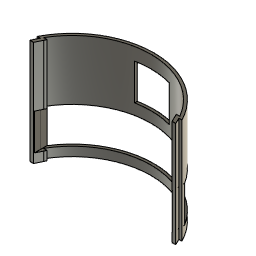
top cap pcb (Autodesk Fusion 360 design; units mm, degrees)
Autodesk Fusion 360 part; units mm, degrees
sketch "Sketch1" plane through (0, 0, 0) normal (0, 0, 1) x (1, 0, 0)
  arc A0 (40, 20.6155) -> (-40, 20.6155) centre (0, 0) ccw
  arc A1 (39.9116, 17.2383) -> (-40.1731, 16.7877) centre (-0.0351, 0.0189) ccw
  line L0 (-40, 20.6155) -> (-38.35, 20.6155)
  line L1 (40, 20.6155) -> (38.2797, 20.6155)
  line L2 (-40.1731, 16.7877) -> (-38.1731, 16.7877)
  line L3 (39.9116, 17.2383) -> (37.9116, 17.2383)
  line L4 (-36.35, 20.6155) -> (-38.1731, 16.7877)
  line L5 (36.2797, 20.6155) -> (37.9116, 17.2383)
  arc A2 (37.5794, 17.9258) -> (37.9116, 17.2383) centre (37.9116, 17.6623) ccw
  line L6 (35.69, 21.8359) -> (39.3471, 21.8359)
  line L7 (35.69, 21.8359) -> (36.2797, 20.6155)
  line L8 (-0.0351, 0.0189) -> (-0.0351, 49.45) construction
  line L9 (-35.7603, 21.8359) -> (-36.35, 20.6155)
  line L10 (-35.7603, 21.8359) -> (-39.4174, 21.8359)
  dimension "d2" = 80
  dimension "d4" = 2
  dimension "d5" = 2
  dimension "d6" = 2
  dimension "d7" = 2
  constraint coincident A1 L0.end
  constraint coincident A1 L1.end
  constraint horizontal L2
  constraint horizontal L3
  constraint coincident L5 A2.start
  constraint tangent L3 A2
  constraint coincident A0 L6.end
  constraint parallel L3 L6
  constraint parallel L5 L7
  constraint coincident A1.centre L8.start
  constraint vertical L8
  constraint symmetric L5.start L8 L4.start
  constraint symmetric L6.start L8 L9.start
  constraint symmetric L6.end L8 L10.end
  measures "d2" distance of A0.end A0.start
  measures "d4" distance of A1.end L2.end
  measures "d5" distance of A1.start L3.end
  measures "d6" distance of L0.end L4.start
  measures "d7" distance of L1.end L5.start
extrude "Extrude1" add sketch "Sketch1" along normal blind 58 contours A0 A1 L1 L6 | A0 A1 L6 L10 | A1 L3 L5 L6 L7 | A0 A1 L0 L10 | A1 L2 L4 L9 L10
sketch "Sketch2" plane through (0, 0, 0) normal (0, 1, 0) x (1, 0, 0)
  line L0 (0, 0) -> (0, -5)
  line L1 (0, -5) -> (38, -5)
  line L2 (38, -5) -> (-38, -5)
  line L3 (-38, -5) -> (-38, -25)
  line L4 (-38, -25) -> (38, -25)
  line L5 (38, -25) -> (38, -5)
  line L6 (-8.3, -51) -> (11.7, -51)
  line L7 (11.7, -51) -> (11.7, -31)
  line L8 (11.7, -31) -> (-8.3, -31)
  line L9 (-8.3, -31) -> (-8.3, -51)
  line L10 (-8.3, -51) -> (11.7, -31) construction
  line L11 (11.7, -51) -> (-8.3, -31) construction
  line L12 (0, -57.95) -> (0, -50.95)
  point P0 (1.7, -41)
  dimension "d10" = 5
  dimension "d11" = 38
  dimension "d12" = 76
  dimension "d13" = 20
  dimension "d14" = 20
  dimension "d15" = 20
  dimension "d16" = 7
  constraint coincident L0.start origin
  constraint vertical L0
  constraint perpendicular L0 L1
  constraint horizontal L2
  constraint vertical L3
  constraint horizontal L4
  constraint vertical L5
  constraint horizontal L6
  constraint perpendicular L6 L7
  constraint parallel L6 L8
  constraint parallel L7 L9
  constraint coincident L10 P0
  constraint coincident L11 P0
  constraint perpendicular L4 L12
  measures "d10" distance of L0.start L0.end
  measures "d11" distance of L0.end L1.end
  measures "d12" distance of L1.end L2.end
  measures "d13" distance of L1.end L4.end
  measures "d14" distance of L7.end L8.end
  measures "d15" distance of L6.end L7.end
  measures "d16" distance of L12.start L12.end
extrude "Extrude2" cut sketch "Sketch2" along normal blind 80
equation "d11 = ( 76 / 2 ) * 1 mm"
